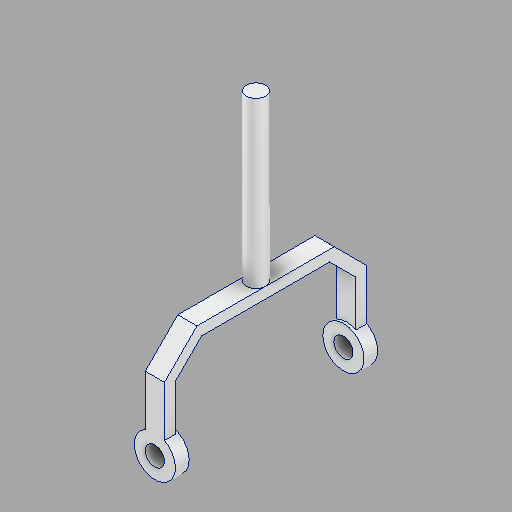
# Autodesk Inventor part: Макет_рамки
Saved by Autodesk Inventor 2025 (Build 290162000, 162)
## iProperties
Created: 2024-11-26
Part Number: Макет_рамки
Material: Алюминий 6061
Document SubType Name: Modeling
Designer: Artem Sannikov
Density: 2.7 g/cm^3
Appearance: Алюминий — плоский
Author: Artem Sannikov
Autodesk Inventor part; units mm, degrees
ref_plane "YZ Plane" through (0, 0, 0) normal (1, 0, 0) x (0, 1, 0)
ref_plane "XZ Plane" through (0, 0, 0) normal (0, 1, 0) x (-1, 0, 0)
ref_plane "XY Plane" through (0, 0, 0) normal (0, 0, 1) x (1, 0, 0)
sketch "Эскиз1" plane through (0, 0, 0) normal (0, 1, 0) x (-1, 0, 0)
  circle A0 centre (0, 0) radius 3.5
  dimension "d0" = 7
  constraints: 1 centre point, 1 coincident
  measures "d0" diameter of A0
extrude "Выдавливание1" add sketch "Эскиз1" along normal blind 60
sketch "Эскиз3" plane through (0, 0, 0) normal (1, 0, 0) x (0, 1, 0)
  line L0 (0, 0) -> (0, -25)
  line L1 (0, -25) -> (-11.8591, -36.8591)
  line L2 (-11.8591, -36.8591) -> (-36.8591, -36.8591)
  line L3 (-36.8591, -32.8591) -> (-13.516, -32.8591)
  line L4 (-13.516, -32.8591) -> (-4, -23.3431)
  line L5 (-4, -23.3431) -> (-4, 0)
  line L6 (-36.8591, -32.8591) -> (-36.8591, -36.8591)
  line L7 (0, 0) -> (-15.7359, 0) construction
  line L8 (0, 0) -> (0, 25)
  line L9 (0, 25) -> (-11.8591, 36.8591)
  line L10 (-11.8591, 36.8591) -> (-36.8591, 36.8591)
  line L11 (-36.8591, 32.8591) -> (-13.516, 32.8591)
  line L12 (-13.516, 32.8591) -> (-4, 23.3431)
  line L13 (-4, 23.3431) -> (-4, 0)
  line L14 (-36.8591, 32.8591) -> (-36.8591, 36.8591)
  dimension "d7" = 25
  dimension "d8" = 45
  dimension "d9" = 25
  dimension "d10" = 4
  constraints: 30 end point, 6 symmetric about line, 2 perpendicular, 2 vertical, 1 horizontal, 2 other
  measures "d7" distance of L0.start L0.end
  measures "d8" angle of L1 L0
  measures "d9" distance of L1.end L2.end
  measures "d10" distance between parallel lines of L2 L3
extrude "Выдавливание3" add sketch "Эскиз3" along normal mid plane 7
sketch "Эскиз4" plane through (3.5, -11.8591, -36.8591) normal (0, 0, -1) x (-1, 0, 0)
  line L0 (7, -25) -> (0, -25) projected
  circle A0 centre (3.5, -25) radius 7.5
  point P0 (3.5, 11.8591)
  dimension "d13" = 15
  constraints: 1 centre point, 1 midpoint
  measures "d13" diameter of A0
extrude "Выдавливание4" add sketch "Эскиз4" against normal blind 5
mirror "Зеркальное отражение1" about plane through (0, 0, 0) normal (0, 0, 1) of "Выдавливание4"
sketch "Эскиз6" plane through (-3.5, -11.8591, 36.8591) normal (0, 0, 1) x (1, 0, 0)
  circle A0 centre (3.5, -25) radius 7.5 projected
  circle A1 centre (3.5, -25) radius 3.5
  point P0 (3.5, 11.8591)
  dimension "d16" = 7
  constraints: 1 centre point, 1 coincident
  measures "d16" diameter of A1
extrude "Выдавливание5" cut sketch "Эскиз6" against normal through all contours A1
